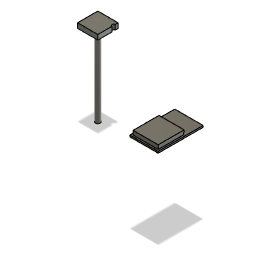
LED_BOX_Grid v3 (Autodesk Fusion 360 design; units mm, degrees)
Autodesk Fusion 360 part; units mm, degrees
sketch "Sketch1" plane through (0, 0, 0) normal (0, 1, 0) x (1, 0, 0)
  line L0 (42.35, 40) -> (42.35, 5.92)
  line L1 (7.27, 40) -> (7.27, 5.92)
  line L2 (7.27, 5.92) -> (16.54, 5.92)
  line L3 (16.54, 5.92) -> (33.08, 5.92)
  line L4 (33.08, 5.92) -> (42.35, 5.92)
  line L5 (9.27, 39) -> (16.54, 39)
  line L6 (16.54, 39) -> (23.81, 39)
  line L7 (25.81, 39) -> (33.08, 39)
  line L8 (16.54, 24.46) -> (23.81, 24.46)
  line L9 (25.81, 24.46) -> (33.08, 24.46)
  line L10 (23.81, 39) -> (23.81, 24.46)
  line L11 (9.27, 39) -> (9.27, 24.46)
  line L12 (9.27, 24.46) -> (16.54, 24.46)
  line L13 (9.27, 22.46) -> (16.54, 22.46)
  line L14 (25.81, 39) -> (25.81, 24.46)
  line L15 (40.35, 39) -> (40.35, 24.46)
  line L16 (33.08, 24.46) -> (40.35, 24.46)
  line L17 (33.08, 39) -> (40.35, 39)
  line L18 (16.54, 22.46) -> (23.81, 22.46)
  line L19 (25.81, 22.46) -> (33.08, 22.46)
  line L20 (33.08, 22.46) -> (40.35, 22.46)
  line L21 (9.27, 7.92) -> (16.54, 7.92)
  line L22 (9.27, 22.46) -> (9.27, 7.92)
  line L23 (16.54, 7.92) -> (23.81, 7.92)
  line L24 (25.81, 7.92) -> (33.08, 7.92)
  line L25 (23.81, 22.46) -> (23.81, 7.92)
  line L26 (25.81, 22.46) -> (25.81, 7.92)
  line L27 (40.35, 22.46) -> (40.35, 7.92)
  line L28 (33.08, 7.92) -> (40.35, 7.92)
  line L29 (7.27, 40) -> (7.27, 41)
  line L30 (42.35, 40) -> (42.35, 41)
  line L31 (7.27, 41) -> (42.35, 41)
  dimension "d40" = 1
  constraint collinear L6 L7
  constraint collinear L8 L9
  constraint collinear L10 L25
  constraint collinear L11 L22
  constraint coincident L19.start L18
  constraint collinear L14 L26
  constraint collinear L15 L27
  constraint collinear L18 L19
  constraint collinear L23 L24
  measures "d40" distance of L0.start L30.end
extrude "Extrude1" add sketch "Sketch1" along normal blind 10 makes body 1
box "BoxPrimitive1" add length 35.08 width 35.08 height 1 placed x (0, 0, -1) y (-1, 0, 0) z (0, 1, 0) at (42.35, 10, -5.92) bodies 1
ref_plane "WorkPlane1" through (24.81, -20, -23.46) normal (0, -1, 0) x (-1, 0, 0)
box "BoxPrimitive2" add length 35.08 width 35.08 height 3 placed x (0, 0, 1) y (-1, 0, 0) z (0, -1, 0) at (42.35, 0, -41) separate body makes body 2
move_body "Move1" bodies 2 to x (1, 0, 0) y (0, 1, 0) z (0, 0, 1) at (0, -22, 0)
copy_body "CopyPasteBodies1" bodies 1 makes body 3
move_body "Move2" bodies 3 to x (1, 0, 0) y (0, 1, 0) z (0, 0, 1) at (-47.0106, 2.1669, 0)
ref_plane "WorkPlane2" through (-22.2006, -2.8331, -23.46) normal (0, -1, 0) x (-1, 0, 0)
sketch "Sketch4" plane through (-22.2006, -2.8331, -23.46) normal (0, -1, 0) x (1, 0, 0)
sketch "Sketch5" plane through (0, 2.1669, 0) normal (0, -1, 0) x (1, 0, 0)
  line L0 (-21.2006, -22.46) -> (-21.2006, -7.92)
  line L1 (-21.2006, -7.92) -> (-6.6606, -7.92)
  line L2 (-6.6606, -7.92) -> (-6.6606, -22.46)
  line L3 (-6.6606, -22.46) -> (-21.2006, -22.46)
  line L4 (-37.7406, -22.46) -> (-37.7406, -7.92)
  line L5 (-37.7406, -7.92) -> (-23.2006, -7.92)
  line L6 (-23.2006, -7.92) -> (-23.2006, -22.46)
  line L7 (-23.2006, -22.46) -> (-37.7406, -22.46)
  line L8 (-21.2006, -39) -> (-21.2006, -24.46)
  line L9 (-21.2006, -24.46) -> (-6.6606, -24.46)
  line L10 (-6.6606, -24.46) -> (-6.6606, -39)
  line L11 (-6.6606, -39) -> (-21.2006, -39)
  line L12 (-37.7406, -39) -> (-37.7406, -24.46)
  line L13 (-37.7406, -24.46) -> (-23.2006, -24.46)
  line L14 (-23.2006, -24.46) -> (-23.2006, -39)
  line L15 (-23.2006, -39) -> (-37.7406, -39)
  line L16 (-39.7406, -5.92) -> (-39.7406, -41)
  line L17 (-39.7406, -41) -> (-4.6606, -41)
  line L18 (-4.6606, -41) -> (-4.6606, -5.92)
  line L19 (-4.6606, -5.92) -> (-39.7406, -5.92)
extrude "Extrude2" add sketch "Sketch5" along normal blind 50 separate body makes body 4
sketch "Sketch6" plane through (0, 2.1669, 0) normal (0, 1, 0) x (-1, 0, 0)
  line L0 (6.6606, -22.46) -> (6.6606, -7.92)
  line L1 (6.6606, -7.92) -> (21.2006, -7.92)
  line L2 (21.2006, -7.92) -> (21.2006, -22.46)
  line L3 (21.2006, -22.46) -> (6.6606, -22.46)
  line L4 (23.2006, -39) -> (23.2006, -24.46)
  line L5 (23.2006, -24.46) -> (37.7406, -24.46)
  line L6 (37.7406, -24.46) -> (37.7406, -39)
  line L7 (37.7406, -39) -> (23.2006, -39)
  line L8 (23.2006, -22.46) -> (23.2006, -7.92)
  line L9 (23.2006, -7.92) -> (37.7406, -7.92)
  line L10 (37.7406, -7.92) -> (37.7406, -22.46)
  line L11 (37.7406, -22.46) -> (23.2006, -22.46)
  line L12 (6.6606, -39) -> (6.6606, -24.46)
  line L13 (6.6606, -24.46) -> (21.2006, -24.46)
  line L14 (21.2006, -24.46) -> (21.2006, -39)
  line L15 (21.2006, -39) -> (6.6606, -39)
  line L16 (39.7406, -5.92) -> (4.6606, -5.92)
  line L17 (4.6606, -5.92) -> (4.6606, -41)
  line L18 (4.6606, -41) -> (39.7406, -41)
  line L19 (39.7406, -41) -> (39.7406, -5.92)
  line L20 (7.6606, -8.92) -> (20.2006, -8.92)
  line L21 (20.2006, -8.92) -> (20.2006, -21.46)
  line L22 (20.2006, -21.46) -> (7.6606, -21.46)
  line L23 (7.6606, -21.46) -> (7.6606, -8.92)
  dimension "d57" = 1
extrude "Extrude3" add sketch "Sketch6" against normal blind 3 separate body contours L20 L21 L22 L23 makes body 5
move_body "Move3" bodies 5 to x (1, 0, 0) y (0, 1, 0) z (0, 0, 1) at (-43.8902, 0, 0.6937)
sketch "Sketch7" plane through (0, -0.8331, 0) normal (0, -1, 0) x (1, 0, 0)
  line L0 (-64.0908, -20.7663) -> (-51.5508, -20.7663)
  line L1 (-51.5508, -20.7663) -> (-51.5508, -8.2263)
  line L2 (-51.5508, -8.2263) -> (-64.0908, -8.2263)
  line L3 (-64.0908, -8.2263) -> (-64.0908, -20.7663)
ref_plane "WorkPlane3" through (-57.8208, -0.8331, -14.4963) normal (0, -1, 0) x (1, 0, 0)
sketch "Sketch8" plane through (-57.8208, -0.8331, -14.4963) normal (0, -1, 0) x (1, 0, 0)
  line L0 (6.27, 6.27) -> (-6.27, 6.27)
  line L1 (-6.27, -6.27) -> (6.27, -6.27)
  line L2 (-6.27, 6.27) -> (-6.27, -6.27)
  line L3 (6.27, -6.27) -> (6.27, 6.27)
  circle A0 centre (0, 0) radius 1.5
  line L4 (-6.27, 0) -> (-1.5, 0)
  line L5 (1.5, 0) -> (6.27, 0)
  line L6 (0, 6.27) -> (0, 1.5)
  line L7 (0, -1.5) -> (0, -6.27)
  dimension "d61" = 3
  constraint midpoint L0 L6.start
  constraint midpoint L1 L7.end
  constraint midpoint L2 L4.start
  constraint midpoint L3 L5.end
  constraint coincident A0 L4.end
  constraint collinear L4 L5
  constraint coincident A0 L5.start
  constraint coincident A0 L6.end
  constraint coincident A0 L7.start
  constraint collinear L6 L7
  measures "d61" diameter of A0
extrude "Extrude4" add sketch "Sketch8" along normal blind 50 contours A0 bodies 5
cylinder "CylinderPrimitive1" cut diameter 2 height -3 placed x (1, 0, 0) y (0, 0, 1) z (0, -1, 0) at (-51.5, -0.8331, -18) bodies 5
box "BoxPrimitive3" add length 27 width 16 height 9 placed x (0, 0, 1) y (1, 0, 0) z (0, 1, 0) at (10, 0, 5) separate body makes body 6
move_face "OffsetFaces1" offset 0.75 5 faces at (15.3333, 0, 14) (10, 3, 23) (15.3333, 9, 14) (15.3333, 3, 32) (26, 3, 23) on bodies 6
shell "Shell1" thickness 1 removed faces 2 at (20.9167, -0.75, 14.25) at (15.0833, 2.75, 5) on bodies 6
sketch "Sketch12" plane through (0, 8.75, 0) normal (0, -1, 0) x (1, 0, 0)
  line L0 (25.75, 31.75) -> (10.25, 31.75)
  line L1 (10.25, 31.75) -> (10.25, 5)
  line L2 (10.25, 5) -> (25.75, 5)
  line L3 (25.75, 5) -> (25.75, 31.75)
  line L4 (10.25, 5) -> (10.25, 5.75)
  line L5 (25.75, 5) -> (25.75, 5.75)
  line L6 (25.75, 5.75) -> (10.25, 5.75)
  dimension "d73" = 0.75
  dimension "d74" = 0.75
  constraint coincident L1.end L2.start
  constraint perpendicular L2 L4
  constraint coincident L2.end L3.start
  constraint perpendicular L2 L5
  measures "d73" distance of L1.end L4.end
  measures "d74" distance of L2.end L5.end
extrude "Extrude5" add sketch "Sketch12" along normal blind 2 contours L1 L2 L3 L4 L5 L6 bodies 6
sketch "Sketch13" plane through (0, -0.75, 0) normal (0, -1, 0) x (1, 0, 0)
  line L0 (10.25, 5) -> (10.25, 31.75)
  line L1 (10.25, 31.75) -> (25.75, 31.75)
  line L2 (25.75, 31.75) -> (25.75, 5)
  line L3 (25.75, 5) -> (26.75, 5)
  line L4 (26.75, 5) -> (26.75, 32.75)
  line L5 (26.75, 32.75) -> (9.25, 32.75)
  line L6 (9.25, 32.75) -> (9.25, 5)
  line L7 (9.25, 5) -> (10.25, 5)
  line L8 (10.25, 5) -> (25.75, 5)
  line L9 (25.75, 5) -> (25.75, 5.75)
  line L10 (25.75, 5.75) -> (10.25, 5.75)
  line L11 (10.25, 5.75) -> (10.25, 5)
  line L12 (9.25, 5) -> (26.75, 5)
  line L13 (26.75, 5) -> (26.75, 32.75)
  line L14 (26.75, 32.75) -> (9.25, 32.75)
  line L15 (9.25, 32.75) -> (9.25, 5)
  constraint coincident L6.end L7.start
  constraint coincident L3.end L4.start
  constraint coincident L4.end L5.start
  constraint coincident L5.end L6.start
extrude "Extrude6" add sketch "Sketch13" along normal blind 1 separate body makes body 7
sketch "Sketch15" plane through (0, -0.75, 0) normal (0, 1, 0) x (-1, 0, 0)
  line L0 (-9.25, 5) -> (-9.25, 32.75)
  line L1 (-9.25, 32.75) -> (-26.75, 32.75)
  line L2 (-26.75, 32.75) -> (-26.75, 5)
  line L3 (-26.75, 5) -> (-9.25, 5)
  line L4 (-10.25, 5) -> (-10.25, 31.75)
  line L5 (-25.75, 31.75) -> (-25.75, 5)
  line L6 (-10.25, 31.75) -> (-25.75, 31.75)
extrude "Extrude7" add sketch "Sketch15" along normal blind 1 contours L3 L4 L5 L6 bodies 7
sketch "Sketch16" plane through (0, 0.25, 0) normal (0, 1, 0) x (-1, 0, 0)
  line L0 (-10.25, 31.75) -> (-25.75, 31.75)
  line L1 (-25.75, 31.75) -> (-25.75, 5)
  line L2 (-25.75, 5) -> (-10.25, 5)
  line L3 (-10.25, 5) -> (-10.25, 31.75)
  line L4 (-25.75, 31.75) -> (-25.75, 15.75)
  line L5 (-25.75, 15.75) -> (-10.25, 15.75)
  dimension "d81" = 16
  constraint coincident L0.end L1.start
  constraint perpendicular L0 L4
  constraint coincident L3 L5.end
  constraint perpendicular L3 L5
  measures "d81" distance of L0.end L4.end
extrude "Extrude8" add sketch "Sketch16" along normal blind 1.5 contours L0 L1 L3 L4 L5 bodies 7
sketch "Sketch17" plane through (10.25, 0, 0) normal (1, 0, 0) x (0, 0, -1)
  line L0 (-5, 6.75) -> (-5.75, 6.75)
  line L1 (-5.75, 6.75) -> (-5.75, 8.75)
  line L2 (-5.75, 8.75) -> (-31.75, 8.75)
  line L3 (-31.75, 8.75) -> (-31.75, -0.75)
  line L4 (-31.75, -0.75) -> (-5, -0.75)
  line L5 (-5, -0.75) -> (-5, 6.75)
  line L6 (-5.75, 6.75) -> (-5.75, -0.75)
  line L7 (-31.75, -0.75, 15.5) -> (-5, -0.75, 15.5)
  line L8 (-5.75, 6.75, 15.5) -> (-5.75, -0.75, 15.5)
  point P0 (-5.75, 6.75)
  constraint coincident P0 L0.end
  constraint coincident L4 L6.end
  constraint perpendicular L4 L6
extrude "Extrude9" add sketch "Sketch17" along normal blind 1 contours L0 L4 L5 L6 bodies 6
sketch "Sketch18" plane through (25.75, 0, 0) normal (-1, 0, 0) x (0, 0, 1)
  line L0 (5.75, 6.75) -> (5, 6.75)
  line L1 (5, 6.75) -> (5, -0.75)
  line L2 (5, -0.75) -> (31.75, -0.75)
  line L3 (31.75, -0.75) -> (31.75, 8.75)
  line L4 (31.75, 8.75) -> (5.75, 8.75)
  line L5 (5.75, 8.75) -> (5.75, 6.75)
  line L6 (5.75, 6.75) -> (5.75, -0.8)
  dimension "d86" = 7.55
  constraint vertical L6
  constraint coincident L0.start L5.end
  measures "d86" distance of L0.start L6.end
extrude "Extrude10" add sketch "Sketch18" along normal blind 1 contours L0 L1 L2 L6 bodies 6
sketch "Sketch19" plane through (0, 0, 32.75) normal (0, 0, 1) x (1, 0, 0)
  line L0 (9.25, 9.75) -> (9.25, -0.75)
  line L1 (9.25, -0.75) -> (26.75, -0.75)
  line L2 (26.75, -0.75) -> (26.75, 9.75)
  line L3 (26.75, 9.75) -> (9.25, 9.75)
  line L4 (26.75, 9.75) -> (18, 9.75)
  line L5 (26.75, -0.75) -> (18, -0.75)
  line L6 (18, 9.75) -> (18, -0.75)
  circle A0 centre (18, 4.5) radius 2
  dimension "d89" = 4
  constraint coincident L2.end L3.start
  constraint midpoint L3 L4.end
  constraint coincident L1.end L2.start
  constraint midpoint L1 L5.end
  constraint midpoint L6 A0.centre
  measures "d89" diameter of A0
extrude "Extrude11" cut sketch "Sketch19" against normal blind 1 contours L6 A0 | L6 A0 bodies 6
sketch "Sketch20" plane through (0, 0, 5) normal (0, 0, -1) x (-1, 0, 0)
  line L0 (-9.25, -0.75) -> (-10.25, -0.75)
  line L1 (-10.25, -0.75) -> (-10.25, 0.25)
  line L2 (-10.25, 0.25) -> (-25.75, 0.25)
  line L3 (-25.75, 0.25) -> (-25.75, -0.75)
  line L4 (-25.75, -0.75) -> (-26.75, -0.75)
  line L5 (-26.75, -0.75) -> (-26.75, -1.75)
  line L6 (-26.75, -1.75) -> (-9.25, -1.75)
  line L7 (-9.25, -1.75) -> (-9.25, -0.75)
  line L8 (-10.25, -0.75) -> (-25.75, -0.75)
  constraint coincident L0.end L1.start
  constraint coincident L3.end L4.start
sketch "Sketch21" plane through (10.25, 0, 0) normal (-1, 0, 0) x (0, 0, 1)
  line L0 (5, -0.75) -> (31.75, -0.75)
  line L1 (31.75, -0.75) -> (31.75, 1.75)
  line L2 (31.75, 1.75) -> (15.75, 1.75)
  line L3 (15.75, 1.75) -> (15.75, 0.25)
  line L4 (15.75, 0.25) -> (5, 0.25)
  line L5 (5, 0.25) -> (5, -0.75)
  line L6 (5, -0.75) -> (7, -0.75)
  line L7 (7, -0.75) -> (7, 0.25)
  dimension "d92" = 2
  dimension "d93" = 1
  constraint coincident L0.start L5.end
  constraint perpendicular L5 L6
  constraint perpendicular L4 L7
  measures "d92" distance of L0.start L6.end
  measures "d93" distance of L6.end L7.end
extrude "Extrude12" cut sketch "Sketch21" against normal blind 1 contours L0 L4 L5 L6 L7 bodies 7
sketch "Sketch22" plane through (25.75, 0, 0) normal (1, 0, 0) x (0, 0, -1)
  line L0 (-31.75, -0.75) -> (-5, -0.75)
  line L1 (-5, -0.75) -> (-5, 0.25)
  line L2 (-5, 0.25) -> (-15.75, 0.25)
  line L3 (-15.75, 0.25) -> (-15.75, 1.75)
  line L4 (-15.75, 1.75) -> (-31.75, 1.75)
  line L5 (-31.75, 1.75) -> (-31.75, -0.75)
  line L6 (-5, -0.75) -> (-7, -0.75)
  line L7 (-7, -0.75) -> (-7, 0.25)
  constraint coincident L0.end L1.start
  constraint coincident L0 L6.end
  constraint perpendicular L1 L6
  constraint coincident L2 L7.end
  constraint perpendicular L2 L7
extrude "Extrude13" cut sketch "Sketch22" against normal blind 1 contours L0 L1 L2 L6 L7 bodies 7
extrude "Extrude14" cut sketch "Sketch20" against normal blind 11 contours L1 L2 L3 L8 bodies 7
hidden bodies 1 2 3 4 6
